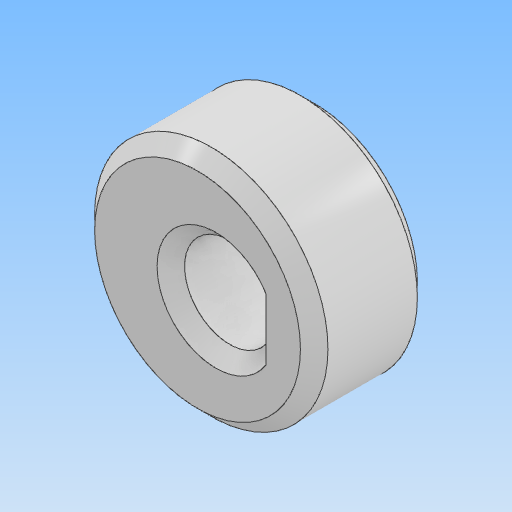
# Autodesk Inventor part: V1_N23Cycloid_AltCam
Saved by Autodesk Inventor 2021 (Build 250183000, 183)
## iProperties
Created: 2021-01-05
Part Number: V1_N23Cycloid_AltCam
Material: PPS Plastic
Document SubType Name: Modeling
Designer: ndevr
Density: 1.637 g/cm^3
Appearance: Smooth - White
Author: ndevr
Autodesk Inventor part; units mm, degrees
ref_plane "YZ Vertical Spine" through (0, 0, 0) normal (1, 0, 0) x (0, 1, 0)
ref_plane "XZ Vertical Span" through (0, 0, 0) normal (0, 1, 0) x (-1, 0, 0)
ref_plane "XY Horizontal" through (0, 0, 0) normal (0, 0, 1) x (1, 0, 0)
derived "V1_N17Cycloid_Cam.ipt"
sketch "Sketch16" plane through (0, 0, 0) normal (0, 0, 1) x (1, 0, 0)
  circle A0 centre (0, 0) radius 6.7333 construction
  circle A1 centre (0, 0) radius 6.7333
  circle A2 centre (-1.0583, 0) radius 2.5
  line L0 (0.9417, 1.5) -> (0.9417, -1.5)
  circle A3 centre (-1.0583, 0) radius 2.6016
  line L1 (1.0433, 1.5335) -> (1.0433, -1.5335)
ref_plane "Top Cycloid Top" through (9.525, 0, 23.6141) normal (0, 0, -1) x (-1, 0, 0)
ref_plane "Cam Center Plane" through (9.525, 0, 16.8672) normal (0, 0, -1) x (-1, 0, 0)
sketch "Sketch2" plane through (0, 0, 0) normal (0, 0, 1) x (1, 0, 0)
  circle A0 centre (-1.0583, 0) radius 2.6016 projected
  line L0 (1.0433, 1.5335) -> (1.0433, -1.5335) projected
  circle A1 centre (0, 0) radius 6.7333 construction
  circle A2 centre (-2.1167, 0) radius 6.7333
  dimension "d1" = 1.0583
  dimension "d2" = 1.0583
  constraints: 1 centre point, 1 equal radius, 1 horizontal alignment
  measures "d1" distance of point (0, 0) A0.centre
  measures "d2" distance of A0.centre A2.centre
extrude "Extrusion1" add sketch "Sketch2" along normal up to surface (6.7469 mm away) from surface at 16.8672 contours A0 L0 | A2 picked at (1.1345, 0.3538)
chamfer "Chamfer1" distance 0.7937 angle 45 6 edges at (-8.85, 0, 23.6141) (-8.85, 0, 16.8672) (-3.6599, 0, 23.6141) (-3.6599, 0, 16.8672) (1.0433, 0, 16.8672) (1.0433, 0, 23.6141)
equation "\"d2\" = d1"
body "Solid1"
